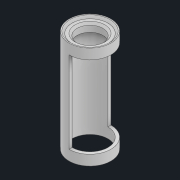
# Autodesk Inventor part: Electronics HousingV2
Saved by Autodesk Inventor 2022.2 (Build 262287000, 287)
## iProperties
Created: 2022-03-22
Part Number: Electronics HousingV2
Material: Generic
Document SubType Name: Modeling
Designer: Michael Lacey
Mass: 6.35033 g
Surface Area: 65.9253 cm^2
Volume: 6.35033 cm^3
Density: 1 g/cm^3
Appearance: Default
Author: Michael Lacey
## iProperties of the stored document Electronics HousingV2_3DPrint.ipt
Created: 2022-03-22
Part Number: Electronics HousingV2_3DPrint
Material: Generic
Document SubType Name: Modeling
Designer: Michael Lacey
Mass: 6.35033 g
Surface Area: 65.9253 cm^2
Volume: 6.35033 cm^3
Density: 1 g/cm^3
Appearance: Default
Author: Michael Lacey
Autodesk Inventor part; units mm, degrees
ref_plane "YZ Plane" through (0, 0, 0) normal (1, 0, 0) x (0, 1, 0)
ref_plane "XZ Plane" through (0, 0, 0) normal (0, 1, 0) x (-1, 0, 0)
ref_plane "XY Plane" through (0, 0, 0) normal (0, 0, 1) x (1, 0, 0)
sketch "Sketch1" plane through (0, 0, 0) normal (0, 1, 0) x (-1, 0, 0)
  circle A0 centre (0, 0) radius 13.0175
  circle A1 centre (0, 0) radius 11.1125
  line L0 (0, 13.0175) -> (0, 11.1125)
  line L1 (0, -11.1125) -> (0, -13.0175)
  circle A2 centre (0, 0) radius 8
  dimension "d0" = 26.035
  dimension "d1" = 22.225
  dimension "d6" = 16
  constraints: 4 end point, 4 point on circle, 3 centre point, 3 coincident, 2 point on line, 1 vertical
  measures "d0" diameter of A0
  measures "d1" diameter of A1
  measures "d6" diameter of A2
extrude "Extrusion1" add sketch "Sketch1" along normal blind 6.35 contours A0 L1 A1 L0 | L0 A1 L1 A0
extrude "Extrusion2" add sketch "Sketch1" against normal blind 25.4 contours A0 L1 A1 L0 picked at (12.2737, -0.9656)
mirror "Mirror1" about plane through (-6.5087, -25.4, 0) normal (0, -1, 0) of "Extrusion2", "Extrusion1"
extrude "Extrusion3" add sketch "Sketch1" along normal blind 5.08 contours A1
chamfer "Chamfer1" distance 1.27 angle 45 2 edges at (11.1125, 6.35, 0) (8, 5.08, 0)
body "Solid1"
